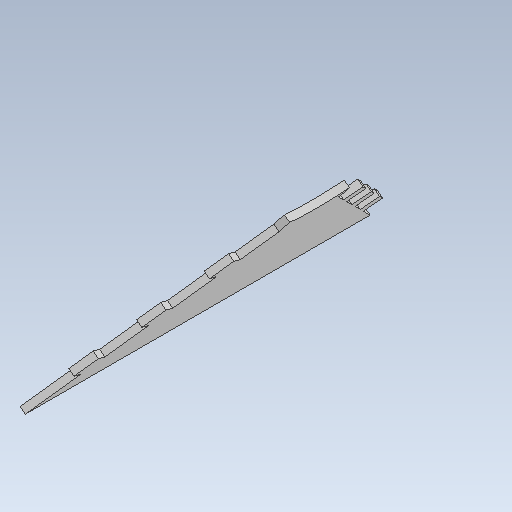
# Autodesk Inventor part: Tolva_Corto
Saved by Autodesk Inventor 2020.1 (Build 241239000, 239)
## iProperties
Created: 2019-12-08
Part Number: Tolva_Corto
Material: Generic
Document SubType Name: Modeling
Designer: Daniel
Density: 1 g/cm^3
Appearance: Default
Author: Daniel
Autodesk Inventor part; units mm, degrees
ref_plane "YZ Plane" through (0, 0, 0) normal (1, 0, 0) x (0, 1, 0)
ref_plane "XZ Plane" through (0, 0, 0) normal (0, 1, 0) x (-1, 0, 0)
sketch "Sketch1" plane through (0, 0, 0) normal (0, 0, 1) x (1, 0, 0)
  line L0 (-27.3641, -15.51) -> (-92.3641, -98.7062)
  line L1 (-26.8641, -15.51) -> (-26.8641, 15.51) projected
  line L2 (-26.8641, -15.51) -> (-27.3641, -15.51) construction
  line L3 (-54.6593, -71.0586) -> (-64.6593, -63.2457)
  point P0 (0, 0)
  dimension "d0" = 0.5
  dimension "d1" = 38
  dimension "d2" = 65
  dimension "d3" = 10
  dimension "d4" = 45
  constraints: 7 end point, 1 horizontal, 1 perpendicular, 1 point on line
  measures "d0" distance from line of L1 L0.start
  measures "d1" angle of L0 L1
  measures "d2" horizontal distance of L0.start L0.end
  measures "d3" horizontal distance of L3.start L3.end
  measures "d4" distance from line of L0.end L3
ref_plane "Work Plane1" through (-64.6593, -63.2457, 0) normal (-0.788, 0.6157, 0) x (-0.6157, -0.788, 0)
sketch "Sketch3" plane through (-64.6593, -63.2457, 0) normal (-0.788, 0.6157, 0) x (-0.6157, -0.788, 0)
  line L0 (25.703, 78.6272) -> (-56.7377, 13.663)
  line L1 (-60.5775, 15.51) -> (-60.5775, 13.663) construction
  line L2 (-56.7377, 13.663) -> (-60.5775, 13.663)
  line L3 (-60.5775, 13.663) -> (-60.5775, 0)
  line L4 (25.703, 78.6272) -> (-56.7377, 13.663)
  line L5 (-56.7377, 13.663) -> (-60.5775, 15.51) construction
  line L6 (-60.5775, 15.51) -> (25.703, 83.5) construction
  line L7 (25.703, 78.6272) -> (25.703, 0)
  line L8 (-89.6466, 0) -> (36.1638, 0) construction
  line L9 (25.703, 83.5) -> (25.703, 78.6272) construction
  line L10 (25.703, -78.6272) -> (-56.7377, -13.663)
  line L11 (-56.7377, -13.663) -> (-60.5775, -13.663)
  line L12 (-60.5775, -13.663) -> (-60.5775, 0)
  line L13 (25.703, -78.6272) -> (25.703, 0)
  point P0 (0, 0)
  constraints: 29 end point, 4 vertical, 3 symmetric about line, 2 horizontal, 1 point on line, 8 other
extrude "Extrusion1" add sketch "Sketch3" along normal blind 3
sketch "Sketch4" plane through (-64.6593, -63.2457, 0) normal (0.788, -0.6157, 0) x (0, 0, -1)
  line L0 (-78.6272, -25.703) -> (-13.663, 56.7377) projected
  line L1 (-23.566, 44.1706) -> (-29.4568, 48.8126)
  line L2 (-29.4568, 48.8126) -> (-35.6462, 40.9582)
  line L3 (-35.6462, 40.9582) -> (-29.7554, 36.3162)
  line L4 (-13.663, 60.5775) -> (13.663, 60.5775) construction
  line L5 (-78.6272, -25.703) -> (-13.663, 56.7377) construction
  line L6 (-52.9764, 18.9659) -> (-47.0856, 14.3238)
  line L7 (-46.787, 26.8203) -> (-52.9764, 18.9659)
  line L8 (-40.8962, 22.1783) -> (-46.787, 26.8203)
  line L9 (-70.3066, -3.0265) -> (-64.4158, -7.6685)
  line L10 (-64.1172, 4.8279) -> (-70.3066, -3.0265)
  line L11 (-58.2264, 0.1859) -> (-64.1172, 4.8279)
  point P0 (0, 89.6466)
  point P1 (-47.0856, 14.3238)
  point P2 (-40.8962, 22.1783)
  dimension "d10" = 7.5
  dimension "d11" = 10
  dimension "d13" = 16
  dimension "d16" = 28
  constraints: 18 end point, 3 perpendicular, 2 point on line, 15 other
  measures "d10" distance of L2.end L3.end
  measures "d11" distance of L1.end L2.end
  measures "d13" distance from line of L0.end L1
  measures "d16" distance of L2.end L6.start
extrude "Extrusion2" add sketch "Sketch4" against normal up to surface (3 mm away)
mirror "Mirror1" about plane through (0, 0, 0) normal (0, 0, 1) of "Extrusion2"
sketch "Sketch6" plane through (-64.6593, -63.2457, 0) normal (0.788, -0.6157, 0) x (0, 0, -1)
  arc A0 (4.4093, 61.3896) -> (-4.4093, 61.3896) centre (0, 89.6466) ccw
  ellipse E0 centre (0, 80.26) end of major axis (0, 60.5775) minor radius 15.51 (4.4093, 61.3896) -> (11.5479, 67.1205) ccw construction
  arc A1 (11.5479, 67.1205) -> (-11.5479, 67.1205) centre (0, 89.6466) ccw construction
  ellipse E1 centre (0, 80.26) end of major axis (0, 60.5775) minor radius 15.51 (-11.5479, 67.1205) -> (-4.4093, 61.3896) ccw construction
  line L0 (-13.663, 56.7377) -> (-13.663, 60.5775) projected
  line L1 (-13.663, 60.5775) -> (-13.663, 64.5225)
  line L2 (13.663, 60.5775) -> (13.663, 56.7377) projected
  line L3 (13.663, 60.5775) -> (13.663, 64.5225)
  circle A2 centre (0, 89.6466) radius 28.5989
  line L4 (-13.663, 60.5775) -> (13.663, 60.5775) projected
  point P0 (0, 89.6466)
  point P1 (4.4093, 61.3896)
  point P2 (-4.4093, 61.3896)
  constraints: 6 point on circle, 4 end point, 3 centre point, 2 collinear, 1 coincident, 1 concentric, 18 other
extrude "Extrusion3" add sketch "Sketch6" against normal up to surface (3 mm away) contours A0 L3 L4 L1 A2
body "Solid1"
